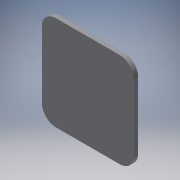
# Autodesk Inventor part: cap
Saved by Autodesk Inventor 2019 (Build 230136000, 136)
## iProperties
Created: 2019-08-20
Part Number: cap
Material: Generic
Document SubType Name: Modeling
Designer: assman
Density: 1 g/cm^3
Appearance: Default
Author: assman
Autodesk Inventor part; units mm, degrees
ref_plane "YZ Plane" through (0, 0, 0) normal (1, 0, 0) x (0, 1, 0)
ref_plane "XZ Plane" through (0, 0, 0) normal (0, 1, 0) x (-1, 0, 0)
ref_plane "XY Plane" through (0, 0, 0) normal (0, 0, 1) x (1, 0, 0)
ref_plane "Work Plane1" through (0, 0, 0) normal (0, 0, 1) x (1, 0, 0)
sketch "Sketch1" plane through (0, 0, 0) normal (0, 0, 1) x (1, 0, 0)
  line L0 (13.075, 9.425) -> (13.075, -9.425) projected
  arc A0 (13.075, 9.425) -> (9.075, 13.425) centre (9.075, 9.425) ccw projected
  line L1 (5, 13.425) -> (9.075, 13.425) projected
  line L2 (-4, 13.425) -> (4, 13.425) projected
  line L3 (5, 13.425) -> (4, 13.425) projected
  line L4 (-4, 13.425) -> (-5, 13.425) projected
  line L5 (-9.075, 13.425) -> (-5, 13.425) projected
  arc A1 (-9.075, 13.425) -> (-13.075, 9.425) centre (-9.075, 9.425) ccw projected
  line L6 (-13.075, -9.425) -> (-13.075, 9.425) projected
  arc A2 (-13.075, -9.425) -> (-9.075, -13.425) centre (-9.075, -9.425) ccw projected
  line L7 (9.075, -13.425) -> (-9.075, -13.425) projected
  arc A3 (9.075, -13.425) -> (13.075, -9.425) centre (9.075, -9.425) ccw projected
  point P0 (0, 0)
extrude "Extrusion1" add sketch "Sketch1" along normal blind 1.2
sketch "Sketch2" plane through (0, 0, 1.2) normal (0, 0, 1) x (1, 0, 0)
  circle A0 centre (0, 0) radius 3.85
  constraints: 1 centre point
extrude "Extrusion2" cut sketch "Sketch2" against normal blind 1.2
sketch "Sketch3" plane through (0, 0, 0) normal (0, 0, -1) x (-1, 0, 0)
  arc A0 (-9.075, 12.225) -> (-11.875, 9.425) centre (-9.075, 9.425) ccw projected
  line L0 (-9.075, 12.225) -> (-5, 12.225) projected
  line L1 (-11.875, -9.425) -> (-11.875, 9.425) projected
  arc A1 (-11.875, -9.425) -> (-9.075, -12.225) centre (-9.075, -9.425) ccw projected
  line L2 (9.075, -12.225) -> (-9.075, -12.225) projected
  arc A2 (9.075, -12.225) -> (11.875, -9.425) centre (9.075, -9.425) ccw projected
  line L3 (11.875, 9.425) -> (11.875, -9.425) projected
  arc A3 (11.875, 9.425) -> (9.075, 12.225) centre (9.075, 9.425) ccw projected
  line L4 (5, 12.225) -> (9.075, 12.225) projected
  line L5 (5, 12.025) -> (9.075, 12.025)
  arc A4 (11.675, 9.425) -> (9.075, 12.025) centre (9.075, 9.425) ccw
  line L6 (11.675, 9.425) -> (11.675, -9.425)
  arc A5 (9.075, -12.025) -> (11.675, -9.425) centre (9.075, -9.425) ccw
  line L7 (9.075, -12.025) -> (-9.075, -12.025)
  arc A6 (-11.675, -9.425) -> (-9.075, -12.025) centre (-9.075, -9.425) ccw
  line L8 (-11.675, -9.425) -> (-11.675, 9.425)
  arc A7 (-9.075, 12.025) -> (-11.675, 9.425) centre (-9.075, 9.425) ccw
  line L9 (-9.075, 12.025) -> (-5, 12.025)
  line L10 (5, 11.525) -> (9.075, 11.525)
  arc A8 (11.175, 9.425) -> (9.075, 11.525) centre (9.075, 9.425) ccw
  line L11 (11.175, 9.425) -> (11.175, -9.425)
  arc A9 (9.075, -11.525) -> (11.175, -9.425) centre (9.075, -9.425) ccw
  line L12 (9.075, -11.525) -> (-9.075, -11.525)
  arc A10 (-11.175, -9.425) -> (-9.075, -11.525) centre (-9.075, -9.425) ccw
  line L13 (-11.175, -9.425) -> (-11.175, 9.425)
  arc A11 (-9.075, 11.525) -> (-11.175, 9.425) centre (-9.075, 9.425) ccw
  line L14 (-9.075, 11.525) -> (-5, 11.525)
  line L15 (-5, 12.025) -> (-5, 11.525)
  line L16 (5, 12.025) -> (5, 11.525)
  point P0 (0, 0)
  dimension "d5" = 0.2
  dimension "d6" = 0.5
  constraints: 24 end point, 16 point on circle, 8 centre point, 1 parallel, 1 vertical, 16 other
  measures "d5" radial gap between concentric circles of A0 A7
  measures "d6" radial gap between concentric circles of A7 A11
extrude "Extrusion3" add sketch "Sketch3" along normal blind 5
body "Solid1"
